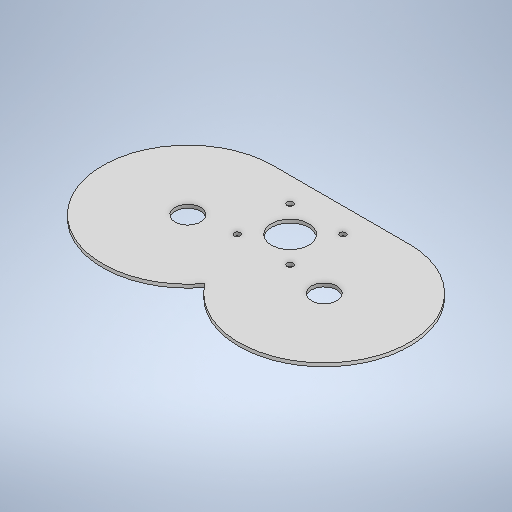
# Autodesk Inventor part: Extruder Frame
Saved by Autodesk Inventor 2025.2 (Build 292293000, 293)
## iProperties
Created: 2025-06-23
Part Number: Extruder Frame
Material: Generic
Document SubType Name: Modeling
Designer: Simon
Density: 1 g/cm^3
Appearance: Default
Author: Simon
Autodesk Inventor part; units mm, degrees
ref_plane "YZ Plane" through (0, 0, 0) normal (1, 0, 0) x (0, 1, 0)
ref_plane "XZ Plane" through (0, 0, 0) normal (0, 1, 0) x (-1, 0, 0)
ref_plane "XY Plane" through (0, 0, 0) normal (0, 0, 1) x (1, 0, 0)
sketch "Sketch1" plane through (0, 0, 0) normal (0, 1, 0) x (-1, 0, 0)
  line L0 (40, 0) -> (-40, 0)
  circle A0 centre (-40, 0) radius 7.5
  circle A1 centre (40, 0) radius 7.5
  circle A2 centre (40, 0) radius 50
  circle A3 centre (-40, 0) radius 50
  line L1 (40, -50) -> (-40, -50)
  line L2 (0, -50) -> (0, -35.5)
  line L3 (15.5, -35.5) -> (-15.5, -35.5)
  line L4 (15.5, -35.5) -> (-15.5, -35.5)
  line L5 (-15.5, -35.5) -> (-15.5, -4.5)
  line L6 (-15.5, -4.5) -> (15.5, -4.5)
  line L7 (15.5, -4.5) -> (15.5, -35.5)
  circle A4 centre (15.5, -35.5) radius 1.8
  circle A5 centre (-15.5, -35.5) radius 1.8
  circle A6 centre (-15.5, -4.5) radius 1.8
  circle A7 centre (15.5, -4.5) radius 1.8
  line L8 (15.5, -35.5) -> (-15.5, -4.5)
  line L9 (-15.5, -4.5) -> (-15.5, -35.5)
  line L10 (-15.5, -35.5) -> (15.5, -4.5)
  circle A8 centre (0, -20) radius 11
  point P0 (0, 0)
  point P1 (0, 30)
  dimension "d3" = 100
  dimension "d4" = 100
  dimension "d0" = 80
  dimension "d1" = 15
  dimension "d2" = 15
  dimension "d5" = 14.5
  dimension "d6" = 31
  dimension "d7" = 31
  dimension "d8" = 3.6
  dimension "d9" = 3.6
  dimension "d10" = 3.6
  dimension "d11" = 3.6
  dimension "d14" = 22
  constraints: 22 end point, 8 coincident, 7 centre point, 5 horizontal, 4 midpoint, 2 parallel, 2 perpendicular, 2 vertical, 6 other
  measures "d0" distance of L0.start L0.end
  measures "d1" diameter of A0
  measures "d2" diameter of A1
  measures "d5" distance of L2.start L2.end
  measures "d6" distance of L3.start L3.end
  measures "d7" distance of L4.end L5.end
  measures "d8" diameter of A4
  measures "d9" diameter of A5
  measures "d10" diameter of A6
  measures "d11" diameter of A7
  measures "d14" diameter of A8
extrude "Extrusion1" add sketch "Sketch1" along normal blind 2 contours A3 L6 A2 L0 | L0 A2 A3 | A3 A2 L3 A4 L7 A7 L6 | A2 L6 A6 L5 A5 L3 A3 | L6 A7 L10 A3 | A3 L10 A8 L8 A2 L6 | A2 L8 A6 L6 | A3 L3 L2 L1 | L10 A7 L7 A4 L8 A8 A3 | A3 A8 L10 | L8 A8 A2 | A2 A8 L10 A5 L5 A6 L8 | L1 L2 L3 A2 | L3 A5 L10 A8 A3 | A3 A8 A2 L3 | A2 A8 L8 A4 L3
body "Solid1"
